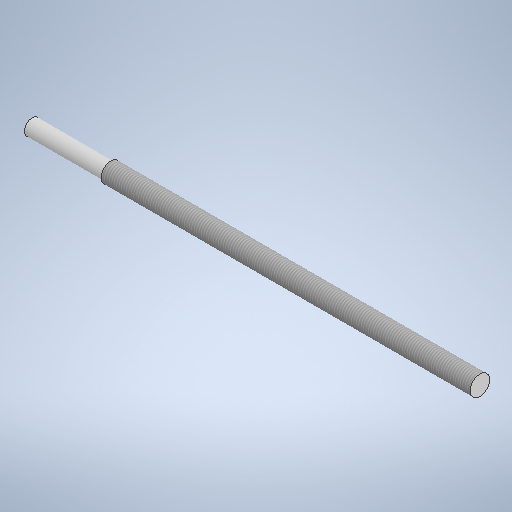
# Autodesk Inventor part: driveshaft2
Saved by Autodesk Inventor 2025.1 (Build 291241000, 241)
## iProperties
Created: 2025-11-11
Part Number: driveshaft2
Material: Generic
Document SubType Name: Modeling
Designer: mukund
Density: 1 g/cm^3
Appearance: Default
Author: mukund
Autodesk Inventor part; units mm, degrees
ref_plane "YZ Plane" through (0, 0, 0) normal (1, 0, 0) x (0, 1, 0)
ref_plane "XZ Plane" through (0, 0, 0) normal (0, 1, 0) x (-1, 0, 0)
ref_plane "XY Plane" through (0, 0, 0) normal (0, 0, 1) x (1, 0, 0)
sketch "Sketch1" plane through (0, 0, 0) normal (1, 0, 0) x (0, 1, 0)
  circle A0 centre (0, 0) radius 6.35
  circle A1 centre (0, 0) radius 8
  dimension "d0" = 12.7
  dimension "d1" = 16
  constraints: 2 centre point, 2 coincident
  measures "d0" diameter of A0
  measures "d1" diameter of A1
extrude "Extrusion1" add sketch "Sketch1" against normal blind 370 contours A0
extrude "Extrusion2" add sketch "Sketch1" against normal blind 305
thread "Thread1" size "M16x2" class "6g" standard "ANSI Metric M Profile" full length
body "Solid1"
